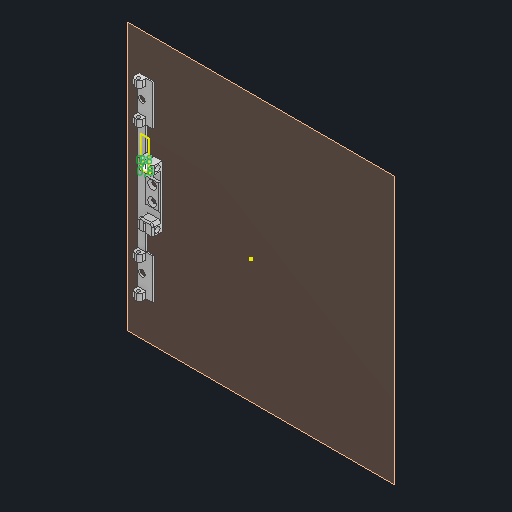
# Autodesk Inventor part: plugassholder
Saved by Autodesk Inventor 2026.2 (Build 302298010, 298A)
## iProperties
Created: 2026-09-27
Part Number: plugassholder
Material: Generic
Document SubType Name: Modeling
Designer: karol
Density: 1 g/cm^3
Appearance: Default
Author: karol
Autodesk Inventor part; units mm, degrees
ref_plane "YZ Plane" through (0, 0, 0) normal (1, 0, 0) x (0, 1, 0)
ref_plane "XZ Plane" through (0, 0, 0) normal (0, 1, 0) x (-1, 0, 0)
ref_plane "XY Plane" through (0, 0, 0) normal (0, 0, 1) x (1, 0, 0)
sketch "Sketch1" plane through (0, 0, 0) normal (0, 0, 1) x (1, 0, 0)
  line L0 (-76, -39.25) -> (-82, -39.25) projected
  line L1 (-82, -39.25) -> (-82, -20.75) projected
  line L2 (-82, -20.75) -> (-76, -20.75) projected
  line L3 (-76, -20.75) -> (-76, -39.25) projected
  line L4 (-76, 20.75) -> (-82, 20.75) projected
  line L5 (-82, 20.75) -> (-82, 39.25) projected
  line L6 (-82, 39.25) -> (-76, 39.25) projected
  line L7 (-76, 39.25) -> (-76, 20.75) projected
  circle A0 centre (-63, -65) radius 1.5 projected
  circle A1 centre (-16.6, -87) radius 1.5 projected
  circle A2 centre (49.6, -87) radius 1.5 projected
  circle A3 centre (46.6, -60) radius 1.5 projected
  circle A4 centre (87, -63) radius 1.5 projected
  circle A5 centre (46.6, -32) radius 1.5 projected
  circle A6 centre (46.6, 32) radius 1.5 projected
  circle A7 centre (87, 63) radius 1.5 projected
  circle A8 centre (46.6, 60) radius 1.5 projected
  circle A9 centre (49.6, 87) radius 1.5 projected
  circle A10 centre (-16.6, 87) radius 1.5 projected
  circle A11 centre (-16.6, 65) radius 1.5 projected
  circle A12 centre (-63, 65) radius 1.5 projected
  line L8 (-58, -60) -> (-60, -60) projected
  line L9 (-60, -60) -> (-60, -39.5) projected
  line L10 (-60, -39.5) -> (-58, -39.5) projected
  line L11 (-58, -39.5) -> (-58, -60) projected
  line L12 (49.6, 30) -> (51.6, 30) projected
  line L13 (51.6, 30) -> (51.6, 9.5) projected
  line L14 (51.6, 9.5) -> (49.6, 9.5) projected
  line L15 (49.6, 9.5) -> (49.6, 30) projected
  line L16 (-58, 39.5) -> (-60, 39.5) projected
  line L17 (-60, 39.5) -> (-60, 60) projected
  line L18 (-60, 60) -> (-58, 60) projected
  line L19 (-58, 60) -> (-58, 39.5) projected
  line L20 (-21.6, -39.5) -> (-19.6, -39.5) projected
  line L21 (-19.6, -39.5) -> (-19.6, -60) projected
  line L22 (-19.6, -60) -> (-21.6, -60) projected
  line L23 (-21.6, -60) -> (-21.6, -39.5) projected
  line L24 (51.6, -30) -> (49.6, -30) projected
  line L25 (49.6, -30) -> (49.6, -9.5) projected
  line L26 (49.6, -9.5) -> (51.6, -9.5) projected
  line L27 (51.6, -9.5) -> (51.6, -30) projected
  line L28 (-21.6, 60) -> (-19.6, 60) projected
  line L29 (-19.6, 60) -> (-19.6, 39.5) projected
  line L30 (-19.6, 39.5) -> (-21.6, 39.5) projected
  line L31 (-21.6, 39.5) -> (-21.6, 60) projected
  line L32 (90, -35) -> (90, 35) projected
  line L33 (90, 35) -> (49.6, 35) projected
  line L34 (49.6, 35) -> (49.6, 60) projected
  line L35 (49.6, 60) -> (90, 60) projected
  line L36 (90, 60) -> (90, 90) projected
  line L37 (90, 90) -> (-19.6, 90) projected
  line L38 (-19.6, 90) -> (-19.6, 65) projected
  line L39 (-19.6, 65) -> (-60, 65) projected
  line L40 (-60, 65) -> (-60, 90) projected
  line L41 (-60, 90) -> (-90, 90) projected
  line L42 (-90, 90) -> (-90, -90) projected
  line L43 (-90, -90) -> (-60, -90) projected
  line L44 (-60, -90) -> (-60, -65) projected
  line L45 (-60, -65) -> (-19.6, -65) projected
  line L46 (-19.6, -65) -> (-19.6, -90) projected
  line L47 (-19.6, -90) -> (90, -90) projected
  line L48 (90, -90) -> (90, -60) projected
  line L49 (90, -60) -> (49.6, -60) projected
  line L50 (49.6, -60) -> (49.6, -35) projected
  line L51 (49.6, -35) -> (90, -35) projected
  line L52 (86, -32) -> (73.8, -32) projected
  line L53 (73.8, -32) -> (73.8, -7.5) projected
  line L54 (73.8, -7.5) -> (86, -7.5) projected
  line L55 (86, -7.5) -> (86, -32) projected
  line L56 (65.8, -32) -> (53.6, -32) projected
  line L57 (53.6, -32) -> (53.6, -7.5) projected
  line L58 (53.6, -7.5) -> (65.8, -7.5) projected
  line L59 (65.8, -7.5) -> (65.8, -32) projected
  line L60 (86, -86) -> (70.6, -86) projected
  line L61 (70.6, -86) -> (70.6, -69.8) projected
  line L62 (70.6, -69.8) -> (86, -69.8) projected
  line L63 (86, -69.8) -> (86, -86) projected
  line L64 (86, 86) -> (86, 69.8) projected
  line L65 (86, 69.8) -> (70.6, 69.8) projected
  line L66 (70.6, 69.8) -> (70.6, 86) projected
  line L67 (70.6, 86) -> (86, 86) projected
  line L68 (73.8, 32) -> (86, 32) projected
  line L69 (86, 32) -> (86, 7.5) projected
  line L70 (86, 7.5) -> (73.8, 7.5) projected
  line L71 (73.8, 7.5) -> (73.8, 32) projected
  line L72 (65.8, 32) -> (65.8, 7.5) projected
  line L73 (65.8, 7.5) -> (53.6, 7.5) projected
  line L74 (53.6, 7.5) -> (53.6, 32) projected
  line L75 (53.6, 32) -> (65.8, 32) projected
  line L76 (-69.6, -87) -> (-85, -87) projected
  line L77 (-85, -87) -> (-85, -70.8) projected
  line L78 (-85, -70.8) -> (-69.6, -70.8) projected
  line L79 (-69.6, -70.8) -> (-69.6, -87) projected
  line L80 (-56, -62) -> (-56, -37.5) projected
  line L81 (-56, -37.5) -> (-43.8, -37.5) projected
  line L82 (-43.8, -37.5) -> (-43.8, -62) projected
  line L83 (-43.8, -62) -> (-56, -62) projected
  line L84 (-56, 62) -> (-43.8, 62) projected
  line L85 (-43.8, 62) -> (-43.8, 37.5) projected
  line L86 (-43.8, 37.5) -> (-56, 37.5) projected
  line L87 (-56, 37.5) -> (-56, 62) projected
  line L88 (-23.6, 62) -> (-23.6, 37.5) projected
  line L89 (-23.6, 37.5) -> (-35.8, 37.5) projected
  line L90 (-35.8, 37.5) -> (-35.8, 62) projected
  line L91 (-35.8, 62) -> (-23.6, 62) projected
  line L92 (-23.6, -62) -> (-35.8, -62) projected
  line L93 (-35.8, -62) -> (-35.8, -37.5) projected
  line L94 (-35.8, -37.5) -> (-23.6, -37.5) projected
  line L95 (-23.6, -37.5) -> (-23.6, -62) projected
  line L96 (-85, 87) -> (-69.6, 87) projected
  line L97 (-69.6, 87) -> (-69.6, 70.8) projected
  line L98 (-69.6, 70.8) -> (-85, 70.8) projected
  line L99 (-85, 70.8) -> (-85, 87) projected
  line L100 (-90, 70.8) -> (-84, 70.8)
  line L101 (-84, 70.8) -> (-84, -70.8)
  line L102 (-84, -70.8) -> (-90, -70.8)
  line L103 (-90, -70.8) -> (-90, 70.8)
  line L104 (-84, -70.8) -> (-90, -70.8)
  line L105 (-90, -70.8) -> (-90, -65.8)
  line L106 (-90, -65.8) -> (-84, -65.8)
  line L107 (-84, -65.8) -> (-84, -70.8)
  line L108 (-84, -65.8) -> (-90, -65.8)
  line L109 (-90, -65.8) -> (-90, -45.8)
  line L110 (-90, -45.8) -> (-84, -45.8)
  line L111 (-84, -45.8) -> (-84, -65.8)
  line L112 (-84, -45.8) -> (-90, -45.8)
  line L113 (-90, -45.8) -> (-90, -40.8)
  line L114 (-90, -40.8) -> (-84, -40.8)
  line L115 (-84, -40.8) -> (-84, -45.8)
  line L116 (-90, 0) -> (-84, 0)
  line L117 (-84, 70.8) -> (-90, 70.8)
  line L118 (-84, 70.8) -> (-90, 70.8)
  line L119 (-90, 70.8) -> (-90, 65.8)
  line L120 (-90, 65.8) -> (-84, 65.8)
  line L121 (-84, 65.8) -> (-84, 70.8)
  line L122 (-84, 65.8) -> (-90, 65.8)
  line L123 (-90, 65.8) -> (-90, 45.8)
  line L124 (-90, 45.8) -> (-84, 45.8)
  line L125 (-84, 45.8) -> (-84, 65.8)
  line L126 (-84, 45.8) -> (-90, 45.8)
  line L127 (-90, 45.8) -> (-90, 40.8)
  line L128 (-90, 40.8) -> (-84, 40.8)
  line L129 (-84, 40.8) -> (-84, 45.8)
  circle A13 centre (-87, 55.8) radius 1.25 projected
  circle A14 centre (-87, -55.8) radius 1.25 projected
  point P0 (0, 0)
  point P1 (-87, -70.8)
  point P2 (-87, 70.8)
  dimension "d0" = 6
  dimension "d1" = 6
  dimension "d2" = 5
  dimension "d3" = 20
  dimension "d4" = 6
  dimension "d5" = 5
  dimension "d6" = 0
  constraints: 60 end point, 13 symmetric about line, 8 parallel, 4 horizontal, 4 perpendicular, 4 point on line, 3 midpoint
  measures "d0" distance of L101.end L102.end
  measures "d1" distance of L105.end L106.end
  measures "d2" distance of L104.end L105.end
  measures "d3" distance of L108.end L109.end
  measures "d4" distance of L113.end L114.end
  measures "d5" distance of L112.end L113.end
  measures "d6" distance from line of point (-87, -70.8) L104
extrude "Extrusion1" add sketch "Sketch1" along normal blind 5.8 contours L42 L106 L101 L78 L102 | L100 L98 L101 L120 L42 | L42 L114 L101 L110 | L124 L101 L128 L42
ref_plane "Work Plane1" through (0, 0, 0) normal (0, 0, 1) x (1, 0, 0)
sketch "Sketch2" plane through (0, 0, 0) normal (0, 0, 1) x (1, 0, 0)
  line L0 (-84, 40.8) -> (-84, 45.8) projected
  line L1 (-84, 45.8) -> (-90, 45.8) projected
  line L2 (-90, 45.8) -> (-90, 40.8) projected
  line L3 (-90, 40.8) -> (-84, 40.8) projected
  line L4 (-90, -40.8) -> (-90, -45.8) projected
  line L5 (-90, -45.8) -> (-84, -45.8) projected
  line L6 (-84, -45.8) -> (-84, -40.8) projected
  line L7 (-84, -40.8) -> (-90, -40.8) projected
  line L8 (-84, 65.8) -> (-84, 70.8) projected
  line L9 (-84, 70.8) -> (-90, 70.8) projected
  line L10 (-90, 70.8) -> (-90, 65.8) projected
  line L11 (-90, 65.8) -> (-84, 65.8) projected
  line L12 (-90, -65.8) -> (-90, -70.8) projected
  line L13 (-90, -70.8) -> (-84, -70.8) projected
  line L14 (-84, -70.8) -> (-84, -65.8) projected
  line L15 (-84, -65.8) -> (-90, -65.8) projected
  line L16 (-84, -65.8) -> (-90, -65.8)
  line L17 (-90, -65.8) -> (-90, -45.8)
  line L18 (-90, -45.8) -> (-84, -45.8)
  line L19 (-84, -45.8) -> (-84, -65.8)
  line L20 (-90, -40.8) -> (-84, -40.8)
  line L21 (-84, -40.8) -> (-84, 40.8)
  line L22 (-84, 40.8) -> (-90, 40.8)
  line L23 (-90, 40.8) -> (-90, -40.8)
  line L24 (-90, 65.8) -> (-84, 65.8)
  line L25 (-84, 65.8) -> (-84, 45.8)
  line L26 (-84, 45.8) -> (-90, 45.8)
  line L27 (-90, 45.8) -> (-90, 65.8)
  point P0 (0, 0)
  constraints: 24 end point, 6 parallel, 3 horizontal, 3 perpendicular
extrude "Extrusion2" add sketch "Sketch2" along normal blind 1 contours L21 L7 L23 L3 | L1 L27 L11 L25 | L19 L15 L17 L5
fillet "Fillet1" radius 2.5 8 edges at (-84, -68.3, 5.8) (-90, -68.3, 5.8) (-90, -43.3, 5.8) (-84, -43.3, 5.8) (-84, 43.3, 5.8) (-90, 43.3, 5.8) (-90, 68.3, 5.8) (-84, 68.3, 5.8)
sketch "Sketch3" plane through (-90, -70.8, 0) normal (0, -1, 0) x (1, 0, 0)
  circle A0 centre (3, 3.6) radius 1.2
  line L0 (6, 0) -> (6, 3.3) projected
  line L1 (0, 0) -> (6, 0) projected
  point P0 (90, 0)
  dimension "d12" = 2.4
  dimension "d13" = 3
  dimension "d14" = 3.6
  constraints: 1 centre point
  measures "d12" diameter of A0
  measures "d13" distance from line of L0 A0.centre
  measures "d14" distance from line of L1 A0.centre
extrude "Extrusion3" cut sketch "Sketch3" against normal blind 5
sketch "Sketch4" plane through (-90, -45.8, 1) normal (0, -1, 0) x (1, 0, 0)
  circle A0 centre (3, 2.6) radius 1.2 projected
  point P0 (90, -1)
extrude "Extrusion4" cut sketch "Sketch4" against normal blind 5
sketch "Sketch5" plane through (-90, 40.8, 1) normal (0, -1, 0) x (1, 0, 0)
  circle A0 centre (3, 2.6) radius 1.2 projected
  point P0 (90, -1)
extrude "Extrusion5" cut sketch "Sketch5" against normal blind 5
sketch "Sketch6" plane through (-90, 65.8, 1) normal (0, -1, 0) x (1, 0, 0)
  circle A0 centre (3, 2.6) radius 1.2 projected
  point P0 (90, -1)
extrude "Extrusion6" cut sketch "Sketch6" against normal blind 5
sketch "Sketch7" plane through (0, 0, 1) normal (0, 0, 1) x (1, 0, 0)
  line L0 (-84, 70.8) -> (-90, 70.8) projected
  line L1 (-84, 70.8) -> (-79, 70.8)
  line L2 (-79, 70.8) -> (-79, 40.8)
  line L3 (-79, 40.8) -> (-84, 40.8)
  line L4 (-84, 40.8) -> (-84, 70.8)
  line L5 (-84, -70.7158) -> (-79, -70.7158)
  line L6 (-79, -70.7158) -> (-79, -40.7158)
  line L7 (-79, -40.7158) -> (-84, -40.7158)
  line L8 (-84, -40.7158) -> (-84, -70.7158)
  point P0 (0, 0)
  dimension "d23" = 5
  dimension "d24" = 30
  dimension "d25" = 5
  dimension "d26" = 30
  constraints: 16 end point, 4 parallel, 2 horizontal, 2 perpendicular, 1 point on line
  measures "d23" distance of L2.end L3.end
  measures "d24" distance of L1.end L2.end
  measures "d25" distance of L7.end L6.end
  measures "d26" distance of L6.end L5.end
extrude "Extrusion7" add sketch "Sketch7" against normal blind 1
sketch "Sketch12" plane through (0, 0, 1) normal (0, 0, 1) x (1, 0, 0)
  line L0 (-84, -40.7158) -> (-84, 40.8) projected
  line L1 (-84, 0.0421) -> (-75, 0.0421)
  line L2 (-75, 0.0421) -> (-75, -9.9579)
  line L3 (-75, -9.9579) -> (-84, -9.9579)
  line L4 (-75, -9.9579) -> (-84, -9.9579)
  line L5 (-84, -9.9579) -> (-84, 10.0421)
  line L6 (-84, 10.0421) -> (-75, 10.0421)
  line L7 (-75, 10.0421) -> (-75, -9.9579)
  point P0 (0, 0)
  dimension "d65" = 9
  dimension "d66" = 10
  dimension "d67" = 20
  constraints: 14 end point, 3 perpendicular, 2 horizontal, 2 parallel, 2 point on line, 1 midpoint
  measures "d65" distance of L1.start L1.end
  measures "d66" distance of L1.end L2.end
  measures "d67" distance of L4.end L5.end
extrude "Extrusion10" add sketch "Sketch12" along normal mid plane 2
sketch "Sketch13" plane through (0, 0, 2) normal (0, 0, 1) x (1, 0, 0)
  circle A0 centre (-78.5, 5.6546) radius 1.65
  circle A1 centre (-78.5, -5.4579) radius 1.65
  line L0 (-75, -9.9579) -> (-75, 10.0421) projected
  line L1 (-75, 10.0421) -> (-84, 10.0421) projected
  line L2 (-84, -9.9579) -> (-75, -9.9579) projected
  point P0 (0, 0)
  point P1 (-79.5, 10.0421)
  point P2 (-79.5, -9.9579)
  dimension "d70" = 3.3
  dimension "d71" = 3.3
  dimension "d72" = 3.5
  dimension "d73" = 4.5
  dimension "d74" = 4.5
  dimension "d75" = 3.5
  constraints: 2 centre point, 2 midpoint
  measures "d70" diameter of A0
  measures "d71" diameter of A1
  measures "d72" distance from line of L0 A0.centre
  measures "d73" distance of point (-79.5, 10.042) A0.centre
  measures "d74" vertical distance of point (-79.5, -9.958) A1.centre
  measures "d75" distance from line of L0 A1.centre
hole "Hole3" at (-78.5, 5.6546, 2) at (-78.5, -5.4579, 2) direction (0, 0, -1) diameter 3.3 depth 2 countersink diameter 6.3 countersink angle 90
sketch "Sketch14" plane through (0, 0, 1) normal (0, 0, 1) x (1, 0, 0)
  line L0 (-76, -39.25) -> (-82, -39.25) projected
  line L1 (-82, -39.25) -> (-82, -20.75) projected
  line L2 (-82, -20.75) -> (-76, -20.75) projected
  line L3 (-76, -20.75) -> (-76, -39.25) projected
  line L4 (-76, 20.75) -> (-82, 20.75) projected
  line L5 (-82, 20.75) -> (-82, 39.25) projected
  line L6 (-82, 39.25) -> (-76, 39.25) projected
  line L7 (-76, 39.25) -> (-76, 20.75) projected
  circle A0 centre (-63, -65) radius 1.5 projected
  circle A1 centre (-16.6, -87) radius 1.5 projected
  circle A2 centre (49.6, -87) radius 1.5 projected
  circle A3 centre (46.6, -60) radius 1.5 projected
  circle A4 centre (87, -63) radius 1.5 projected
  circle A5 centre (46.6, -32) radius 1.5 projected
  circle A6 centre (46.6, 32) radius 1.5 projected
  circle A7 centre (87, 63) radius 1.5 projected
  circle A8 centre (46.6, 60) radius 1.5 projected
  circle A9 centre (49.6, 87) radius 1.5 projected
  circle A10 centre (-16.6, 87) radius 1.5 projected
  circle A11 centre (-16.6, 65) radius 1.5 projected
  circle A12 centre (-63, 65) radius 1.5 projected
  line L8 (-58, -60) -> (-60, -60) projected
  line L9 (-60, -60) -> (-60, -39.5) projected
  line L10 (-60, -39.5) -> (-58, -39.5) projected
  line L11 (-58, -39.5) -> (-58, -60) projected
  line L12 (49.6, 30) -> (51.6, 30) projected
  line L13 (51.6, 30) -> (51.6, 9.5) projected
  line L14 (51.6, 9.5) -> (49.6, 9.5) projected
  line L15 (49.6, 9.5) -> (49.6, 30) projected
  line L16 (-58, 39.5) -> (-60, 39.5) projected
  line L17 (-60, 39.5) -> (-60, 60) projected
  line L18 (-60, 60) -> (-58, 60) projected
  line L19 (-58, 60) -> (-58, 39.5) projected
  line L20 (-21.6, -39.5) -> (-19.6, -39.5) projected
  line L21 (-19.6, -39.5) -> (-19.6, -60) projected
  line L22 (-19.6, -60) -> (-21.6, -60) projected
  line L23 (-21.6, -60) -> (-21.6, -39.5) projected
  line L24 (51.6, -30) -> (49.6, -30) projected
  line L25 (49.6, -30) -> (49.6, -9.5) projected
  line L26 (49.6, -9.5) -> (51.6, -9.5) projected
  line L27 (51.6, -9.5) -> (51.6, -30) projected
  line L28 (-21.6, 60) -> (-19.6, 60) projected
  line L29 (-19.6, 60) -> (-19.6, 39.5) projected
  line L30 (-19.6, 39.5) -> (-21.6, 39.5) projected
  line L31 (-21.6, 39.5) -> (-21.6, 60) projected
  line L32 (90, -35) -> (90, 35) projected
  line L33 (90, 35) -> (49.6, 35) projected
  line L34 (49.6, 35) -> (49.6, 60) projected
  line L35 (49.6, 60) -> (90, 60) projected
  line L36 (90, 60) -> (90, 90) projected
  line L37 (90, 90) -> (-19.6, 90) projected
  line L38 (-19.6, 90) -> (-19.6, 65) projected
  line L39 (-19.6, 65) -> (-60, 65) projected
  line L40 (-60, 65) -> (-60, 90) projected
  line L41 (-60, 90) -> (-90, 90) projected
  line L42 (-90, 90) -> (-90, -90) projected
  line L43 (-90, -90) -> (-60, -90) projected
  line L44 (-60, -90) -> (-60, -65) projected
  line L45 (-60, -65) -> (-19.6, -65) projected
  line L46 (-19.6, -65) -> (-19.6, -90) projected
  line L47 (-19.6, -90) -> (90, -90) projected
  line L48 (90, -90) -> (90, -60) projected
  line L49 (90, -60) -> (49.6, -60) projected
  line L50 (49.6, -60) -> (49.6, -35) projected
  line L51 (49.6, -35) -> (90, -35) projected
  line L52 (86, -32) -> (73.8, -32) projected
  line L53 (73.8, -32) -> (73.8, -7.5) projected
  line L54 (73.8, -7.5) -> (86, -7.5) projected
  line L55 (86, -7.5) -> (86, -32) projected
  line L56 (65.8, -32) -> (53.6, -32) projected
  line L57 (53.6, -32) -> (53.6, -7.5) projected
  line L58 (53.6, -7.5) -> (65.8, -7.5) projected
  line L59 (65.8, -7.5) -> (65.8, -32) projected
  line L60 (86, -86) -> (70.6, -86) projected
  line L61 (70.6, -86) -> (70.6, -69.8) projected
  line L62 (70.6, -69.8) -> (86, -69.8) projected
  line L63 (86, -69.8) -> (86, -86) projected
  line L64 (86, 86) -> (86, 69.8) projected
  line L65 (86, 69.8) -> (70.6, 69.8) projected
  line L66 (70.6, 69.8) -> (70.6, 86) projected
  line L67 (70.6, 86) -> (86, 86) projected
  line L68 (73.8, 32) -> (86, 32) projected
  line L69 (86, 32) -> (86, 7.5) projected
  line L70 (86, 7.5) -> (73.8, 7.5) projected
  line L71 (73.8, 7.5) -> (73.8, 32) projected
  line L72 (65.8, 32) -> (65.8, 7.5) projected
  line L73 (65.8, 7.5) -> (53.6, 7.5) projected
  line L74 (53.6, 7.5) -> (53.6, 32) projected
  line L75 (53.6, 32) -> (65.8, 32) projected
  line L76 (-69.6, -87) -> (-85, -87) projected
  line L77 (-85, -87) -> (-85, -70.8) projected
  line L78 (-85, -70.8) -> (-69.6, -70.8) projected
  line L79 (-69.6, -70.8) -> (-69.6, -87) projected
  line L80 (-56, -62) -> (-56, -37.5) projected
  line L81 (-56, -37.5) -> (-43.8, -37.5) projected
  line L82 (-43.8, -37.5) -> (-43.8, -62) projected
  line L83 (-43.8, -62) -> (-56, -62) projected
  line L84 (-56, 62) -> (-43.8, 62) projected
  line L85 (-43.8, 62) -> (-43.8, 37.5) projected
  line L86 (-43.8, 37.5) -> (-56, 37.5) projected
  line L87 (-56, 37.5) -> (-56, 62) projected
  line L88 (-23.6, 62) -> (-23.6, 37.5) projected
  line L89 (-23.6, 37.5) -> (-35.8, 37.5) projected
  line L90 (-35.8, 37.5) -> (-35.8, 62) projected
  line L91 (-35.8, 62) -> (-23.6, 62) projected
  line L92 (-23.6, -62) -> (-35.8, -62) projected
  line L93 (-35.8, -62) -> (-35.8, -37.5) projected
  line L94 (-35.8, -37.5) -> (-23.6, -37.5) projected
  line L95 (-23.6, -37.5) -> (-23.6, -62) projected
  line L96 (-85, 87) -> (-69.6, 87) projected
  line L97 (-69.6, 87) -> (-69.6, 70.8) projected
  line L98 (-69.6, 70.8) -> (-85, 70.8) projected
  line L99 (-85, 70.8) -> (-85, 87) projected
  line L100 (-84, -40.7158) -> (-84, -9.9579) projected
  line L101 (-84, -20.75) -> (-75, -20.75)
  line L102 (-75, -20.75) -> (-75, -22.75)
  line L103 (-75, -22.75) -> (-84, -22.75)
  line L104 (-84, -22.75) -> (-84, -20.75)
  line L105 (-75, -9.9579) -> (-84, -9.9579) projected
  line L106 (-75, -20.75) -> (-84, -20.75)
  line L107 (-84, -20.75) -> (-84, -9.9579)
  line L108 (-84, -9.9579) -> (-75, -9.9579)
  line L109 (-75, -9.9579) -> (-75, -20.75)
  line L110 (-84, 20.75) -> (-75, 20.75)
  line L111 (-75, 20.75) -> (-75, 22.75)
  line L112 (-75, 22.75) -> (-84, 22.75)
  line L113 (-84, 22.75) -> (-84, 20.75)
  line L114 (-75, 10.0421) -> (-84, 10.0421) projected
  line L115 (-75, 20.75) -> (-84, 20.75)
  line L116 (-84, 20.75) -> (-84, 10.0421)
  line L117 (-84, 10.0421) -> (-75, 10.0421)
  line L118 (-75, 10.0421) -> (-75, 20.75)
  circle A13 centre (-87, 55.8) radius 1.25 projected
  circle A14 centre (-87, -55.8) radius 1.25 projected
  point P0 (0, 0)
  dimension "d83" = 2
  dimension "d84" = 2
  constraints: 32 end point, 8 parallel, 4 horizontal, 4 perpendicular, 3 point on line
  measures "d83" distance of L101.end L102.end
  measures "d84" distance of L111.end L110.end
extrude "Extrusion11" add sketch "Sketch14" against normal blind 1 contours L103 L1 L2 L3 | L3 L101 L102 L103 | L103 L100 L101 L1 | L2 L101 L100 L105 L109 | L110 L118 L114 L116 L4 | L4 L5 L112 L7 | L7 L112 L111 L110 | L110 L113 L112 L5
sketch "Sketch15" plane through (0, 0, 1) normal (0, 0, 1) x (1, 0, 0)
  line L0 (-75, 10.0421) -> (-75, 22.75) projected
  line L1 (-75, 22.75) -> (-82, 22.75)
  line L2 (-82, 22.75) -> (-82, 16.75)
  line L3 (-82, 16.75) -> (-75, 16.75)
  line L4 (-75, 16.75) -> (-75, 22.75)
  line L5 (-75, -22.75) -> (-82, -22.75)
  line L6 (-82, -22.75) -> (-82, -16.75)
  line L7 (-82, -16.75) -> (-75, -16.75)
  line L8 (-75, -16.75) -> (-75, -22.75)
  line L9 (-84, -22.75) -> (-75, -22.75) projected
  point P0 (0, 0)
  dimension "d87" = 7
  dimension "d88" = 6
  dimension "d89" = 6
  constraints: 16 end point, 4 parallel, 2 horizontal, 2 perpendicular, 2 point on line, 1 collinear
  measures "d87" distance of L3.end L2.end
  measures "d88" distance of L2.end L1.end
  measures "d89" distance of L5.end L6.end
extrude "Extrusion12" add sketch "Sketch15" along normal blind 6
sketch "Sketch16" plane through (-82, 16.75, 1) normal (-1, 0, 0) x (0, 0, 1)
  circle A0 centre (2.5, 3) radius 1.65
  line L0 (0, 0) -> (6, 0) projected
  line L1 (-3, 73.25) -> (-3, -106.75) projected
  line L2 (7, 15.25) -> (7, -48.75) projected
  line L3 (0, 24.05) -> (0, -57.55) projected
  point P0 (-1, -16.75)
  dimension "d92" = 3.3
  dimension "d93" = 3
  dimension "d95" = 2.5
  constraints: 1 centre point
  measures "d92" diameter of A0
  measures "d93" distance from line of L0 A0.centre
  measures "d95" distance from line of L3 A0.centre
extrude "Extrusion13" cut sketch "Sketch16" against normal blind 7
sketch "Sketch17" plane through (0, 0, 7) normal (0, 0, 1) x (1, 0, 0)
  line L0 (-82, 16.75) -> (-75, 16.75) projected
  line L1 (-75, 16.75) -> (-75, 22.75) projected
  line L2 (-75, 22.75) -> (-82, 22.75) projected
  line L3 (-82, 22.75) -> (-82, 16.75) projected
  line L4 (-76, 39.25) -> (-76, 20.75) projected
  line L5 (-82, 20.75) -> (-82, 39.25) projected
  line L6 (-82, 39.25) -> (-76, 39.25) projected
  line L7 (-79, 22.75) -> (-79, 16.75)
  line L8 (-82, 16.75) -> (-75, 16.75) projected
  line L9 (-79, 22.75) -> (-78.2, 22.75)
  line L10 (-78.2, 22.75) -> (-78.2, 16.75)
  line L11 (-78.2, 16.75) -> (-79, 16.75)
  line L12 (-79, 16.75) -> (-79, 22.75)
  line L13 (-79, 16.75) -> (-79.8, 16.75)
  line L14 (-79.8, 16.75) -> (-79.8, 22.75)
  line L15 (-79.8, 22.75) -> (-79, 22.75)
  line L16 (-79, 22.75) -> (-79, 16.75)
  point P0 (0, 0)
  dimension "d98" = 3
  dimension "d99" = 0.8
  dimension "d100" = 0.8
  constraints: 18 end point, 4 parallel, 4 point on line, 3 perpendicular, 2 horizontal
  measures "d98" distance between parallel lines of L5 L7
  measures "d99" distance of L10.end L11.end
  measures "d100" distance of L14.end L15.end
sketch "Sketch18" plane through (-84, 22.75, 0) normal (0, 1, 0) x (1, 0, 0)
  line L0 (9, -1) -> (2, -1) projected
  line L1 (5.8, -7) -> (5.2751, -1)
  line L2 (5.8, -7) -> (11.8229, -7) construction
  line L3 (4.2, -7) -> (3.6751, -1)
  line L4 (4.2, -7) -> (10.2229, -7) construction
  line L5 (5.8, -7) -> (4.2, -7)
  line L6 (5.2751, -1) -> (3.6751, -1)
  point P0 (84, 0)
  dimension "d101" = 95
  dimension "d102" = 95
  constraints: 12 end point, 2 collinear, 2 equal length, 2 horizontal, 2 point on line
  measures "d101" angle of L2 L1
  measures "d102" angle of L4 L3
extrude "Extrusion14" cut sketch "Sketch18" against normal blind 6
sketch "Sketch19" plane through (-82, -16.75, 1) normal (0, 1, 0) x (1, 0, 0)
  line L0 (1.6751, 0) -> (3.2751, 0) projected
  line L1 (3.2751, 0) -> (3.8, -6) projected
  line L2 (2.2, -6) -> (1.6751, 0) projected
  line L3 (0, -6) -> (6, -6) projected
  point P0 (82, 1)
extrude "Extrusion15" cut sketch "Sketch19" against normal blind 6
sketch "Sketch20" plane through (-82, -22.75, 1) normal (-1, 0, 0) x (0, 0, 1)
  circle A0 centre (2.5, 3) radius 1.65
  line L0 (0, 63.55) -> (0, -18.05) projected
  line L1 (0, 0) -> (6, 0) projected
  point P0 (-1, 22.75)
  dimension "d107" = 3.3
  dimension "d108" = 2.5
  dimension "d109" = 3
  constraints: 1 centre point
  measures "d107" diameter of A0
  measures "d108" distance from line of L0 A0.centre
  measures "d109" distance from line of L1 A0.centre
extrude "Extrusion16" cut sketch "Sketch20" against normal blind 7
sketch "Sketch21" plane through (-82, -22.75, 1) normal (-1, 0, 0) x (0, 0, 1)
  circle A0 centre (2.5, 3) radius 1.65 projected
  line L0 (0, 0) -> (0, 6) projected
  line L1 (0, 0) -> (6, 0) projected
  line L2 (6, 6) -> (6, 0) projected
  line L3 (0, 6) -> (6, 6) projected
  point P0 (-1, 22.75)
extrude "Extrusion17" add sketch "Sketch21" along normal blind 2
sketch "Sketch22" plane through (-82, 16.75, 1) normal (-1, 0, 0) x (0, 0, 1)
  circle A0 centre (2.5, 3) radius 1.65 projected
  line L0 (0, 0) -> (0, 6) projected
  line L1 (0, 0) -> (6, 0) projected
  line L2 (6, 6) -> (6, 0) projected
  line L3 (0, 6) -> (6, 6) projected
  point P0 (-1, -16.75)
extrude "Extrusion18" add sketch "Sketch22" along normal blind 2
sketch "Sketch23" plane through (-75, -9.9579, 2) normal (1, 0, 0) x (0, 0, -1)
  circle A0 centre (-1.5, -9.7921) radius 1.65 projected
  circle A1 centre (-1.5, -9.7921) radius 2
  circle A2 centre (-1.5, 29.7079) radius 1.65 projected
  circle A3 centre (-1.5, 29.7079) radius 2
  point P0 (2, 9.9579)
  dimension "d116" = 4
  constraints: 2 centre point, 2 coincident
  measures "d116" diameter of A1
extrude "Extrusion19" cut sketch "Sketch23" against normal blind 4 contours A0 | A1 | A2 | A3
sketch "Sketch24" plane through (-75, -9.9579, 2) normal (1, 0, 0) x (0, 0, -1)
  circle A0 centre (-1.5, -9.7921) radius 2 projected
  circle A1 centre (-1.5, 29.7079) radius 2 projected
  line L0 (0, 20) -> (1, 20) projected
  line L1 (0, 0) -> (0, 20) projected
  line L2 (1, 0) -> (0, 0) projected
  line L3 (1, -6.7921) -> (1, 0) projected
  line L4 (1, -6.7921) -> (-5, -6.7921) projected
  line L5 (-5, -12.7921) -> (-5, -6.7921) projected
  line L6 (-5, -12.7921) -> (2, -12.7921) projected
  line L7 (2, 32.7079) -> (2, -12.7921) projected
  line L8 (2, 32.7079) -> (-5, 32.7079) projected
  line L9 (-5, 26.7079) -> (-5, 32.7079) projected
  line L10 (1, 26.7079) -> (-5, 26.7079) projected
  line L11 (1, 20) -> (1, 26.7079) projected
  point P0 (2, 9.9579)
extrude "Extrusion20" add sketch "Sketch24" along normal blind 2
sketch "Sketch25" plane through (-80.3249, 22.75, 1) normal (0, 1, 0) x (1, 0, 0)
  line L0 (1.6, 0) -> (2.1249, -6) projected
  line L1 (2.1249, -6) -> (7.3249, -6) projected
  line L2 (7.3249, 1) -> (7.3249, -6) projected
  line L3 (-3.6751, 1) -> (7.3249, 1) projected
  line L4 (-3.6751, 0) -> (-3.6751, 1) projected
  line L5 (-3.6751, -6) -> (-3.6751, 0) projected
  line L6 (0.5249, -6) -> (-3.6751, -6) projected
  line L7 (0.5249, -6) -> (0, 0) projected
  line L8 (0, 0) -> (1.6, 0) projected
  line L9 (2.1249, -6) -> (1.5125, 1)
  line L10 (0.5249, -6) -> (-0.0875, 1)
  line L11 (1.5125, 1) -> (-0.0875, 1)
  line L12 (1.6, 0) -> (0, 0)
  point P0 (80.3249, 1)
  constraints: 8 end point, 4 point on line, 1 collinear, 1 parallel
extrude "Extrusion21" cut sketch "Sketch25" against normal blind 2 contours L8 L10 L3 L9
sketch "Sketch26" plane through (-80.3249, -22.75, 1) normal (0, -1, 0) x (1, 0, 0)
  line L0 (1.5125, -1) -> (1.6, 0) projected
  line L1 (0, 0) -> (-0.0875, -1) projected
  line L2 (1.6, 0) -> (0, 0) projected
  line L3 (-9.6751, -1) -> (20.3249, -1) projected
  point P0 (80.3249, -1)
extrude "Extrusion22" cut sketch "Sketch26" against normal blind 2
sketch "Sketch27" plane through (0, 0, 1) normal (0, 0, 1) x (1, 0, 0)
  line L0 (-84, -16.75) -> (-80.3249, -16.75) projected
  line L1 (-73, -22.75) -> (-73, 22.75) projected
  line L2 (-84, -16.75) -> (-73, -16.75)
  line L3 (-73, -16.75) -> (-73, -14.75)
  line L4 (-73, -14.75) -> (-84, -14.75)
  line L5 (-84, -14.75) -> (-84, -16.75)
  line L6 (-78.2, 16.75) -> (-73, 16.75) projected
  line L7 (-73, 16.75) -> (-84, 16.75)
  line L8 (-84, 16.75) -> (-84, 14.75)
  line L9 (-84, 14.75) -> (-73, 14.75)
  line L10 (-73, 14.75) -> (-73, 16.75)
  point P0 (0, 0)
  dimension "d125" = 2
  dimension "d126" = 2
  constraints: 16 end point, 4 parallel, 2 horizontal, 2 perpendicular, 1 point on line
  measures "d125" distance of L3.end L2.end
  measures "d126" distance of L8.end L7.end
extrude "Extrusion23" add sketch "Sketch27" along normal blind 6
fillet "Fillet2" radius 2 4 edges at (-84, -14.75, 4) (-84, 14.75, 4) (-73, -14.75, 4) (-73, 14.75, 4)
fillet "Fillet3" radius 1 10 edges at (-78.5, 14.75, 7) (-83.4142, 15.3358, 7) (-84, 19.75, 7) (-73, 19.75, 7) (-73.5858, 15.3358, 7) (-83.4142, -15.3358, 7) (-78.5, -14.75, 7) (-73.5858, -15.3358, 7) (-73, -19.75, 7) (-84, -19.75, 7)
fillet "Fillet4" radius 1 4 edges at (-78.5, 10.0421, 2) (-84, 0.0421, 2) (-78.5, -9.9579, 2) (-73, 0.0421, 2)
sketch "Sketch28" plane through (0, 0, 1) normal (0, 0, 1) x (1, 0, 0)
  circle A0 centre (-87, 55.8) radius 1.65
  line L0 (-87.5, 65.8) -> (-86.5, 65.8) projected
  line L1 (-90, 65.8) -> (-90, 45.8) projected
  circle A1 centre (-87, -55.8) radius 1.65
  line L2 (-87.5, -45.8) -> (-86.5, -45.8) projected
  line L3 (-90, -45.8) -> (-90, -65.8) projected
  point P0 (0, 0)
  point P1 (-87, 65.8)
  point P2 (-90, 55.8)
  point P3 (-87, -45.8)
  dimension "d132" = 3.3
  dimension "d133" = 10
  dimension "d134" = 3
  dimension "d135" = 3.3
  dimension "d136" = 10
  dimension "d137" = 3
  constraints: 3 midpoint, 2 centre point
  measures "d132" diameter of A0
  measures "d133" distance of A0.centre point (-87, 65.8)
  measures "d134" distance of point (-90, 55.8) A0.centre
  measures "d135" diameter of A1
  measures "d136" distance of point (-87, -45.8) A1.centre
  measures "d137" distance from line of L3 A1.centre
extrude "Extrusion24" cut sketch "Sketch28" against normal blind 1
chamfer "Chamfer1" distance 0.7 angle 45 2 edges at (-88.65, -55.8, 1) (-88.65, 55.8, 1)
body "Solid1"
